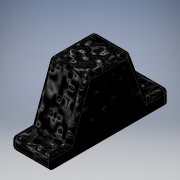
# Autodesk Inventor part: Fuse Block
Saved by Autodesk Inventor 2017 (Build 210142000, 142)
## iProperties
Created: 2017-02-10
Part Number: Fuse Block
Material: Generic
Document SubType Name: Modeling
Designer: michael
Density: 1 g/cm^3
Appearance: Default
Author: michael
Autodesk Inventor part; units mm, degrees
ref_plane "YZ Plane" through (0, 0, 0) normal (1, 0, 0) x (0, 1, 0)
ref_plane "XZ Plane" through (0, 0, 0) normal (0, 1, 0) x (-1, 0, 0)
ref_plane "XY Plane" through (0, 0, 0) normal (0, 0, 1) x (1, 0, 0)
sketch "Sketch1" plane through (0, 0, 0) normal (0, 1, 0) x (-1, 0, 0)
  line L0 (-14.45, 46.075) -> (14.45, 46.075)
  line L1 (14.45, 46.075) -> (14.45, -46.075)
  line L2 (14.45, -46.075) -> (-14.45, -46.075)
  line L3 (-14.45, -46.075) -> (-14.45, 46.075)
  line L4 (-14.45, 46.075) -> (14.45, -46.075) construction
  line L5 (14.45, 46.075) -> (-14.45, -46.075) construction
  point P0 (0, 0)
  dimension "d0" = 28.9
  dimension "d1" = 92.15
  constraints: 12 end point, 2 midpoint, 2 parallel, 1 horizontal, 1 perpendicular
  measures "d0" distance of L1.end L2.end
  measures "d1" distance of L0.end L1.end
extrude "Extrusion1" add sketch "Sketch1" against normal blind 10
sketch "Sketch2" plane through (0, 0, 0) normal (0, 1, 0) x (1, 0, 0)
  point P0 (0, 0)
sketch "Sketch3" plane through (0, 0, 0) normal (0, 1, 0) x (1, 0, 0)
  line L0 (-14.45, -30.5) -> (14.45, -30.5)
  line L1 (14.45, -30.5) -> (14.45, 30.5)
  line L2 (14.45, 30.5) -> (-14.45, 30.5)
  line L3 (-14.45, 30.5) -> (-14.45, -30.5)
  line L4 (-14.45, -30.5) -> (14.45, 30.5) construction
  line L5 (14.45, -30.5) -> (-14.45, 30.5) construction
  point P0 (0, 0)
  dimension "d4" = 28.9
  dimension "d5" = 61
  constraints: 12 end point, 2 midpoint, 2 parallel, 1 horizontal, 1 perpendicular
  measures "d4" distance of L2.end L1.end
  measures "d5" distance of L1.end L0.end
extrude "Extrusion2" add sketch "Sketch3" along normal blind 38
sketch "Sketch4" plane through (0, -10, 0) normal (0, -1, 0) x (1, 0, 0)
  circle A0 centre (0, 39.725) radius 2.7
  circle A1 centre (0, -39.725) radius 2.7
  line L0 (-14.45, -46.075) -> (14.45, -46.075) projected
  line L1 (14.45, -46.075) -> (14.45, 46.075) projected
  point P0 (0, 0)
  dimension "d8" = 5.4
  dimension "d9" = 5.4
  dimension "d10" = 79.45
  dimension "d11" = 6.35
  dimension "d12" = 14.45
  dimension "d13" = 14.45
  constraints: 2 centre point
  measures "d8" diameter of A0
  measures "d9" diameter of A1
  measures "d10" distance of A1.centre A0.centre
  measures "d11" distance from line of L0 A1.centre
  measures "d12" distance from line of L1 A1.centre
  measures "d13" distance from line of L1 A0.centre
hole "Hole1" at (0, -10, -39.725) at (0, -10, 39.725) direction (0, 1, 0) diameter 6.35 end through all
draft "FaceDraft1" angle 20 pull direction (0, 1, 0) faces at (4.8167, 12.6667, -30.5) fixed edges at (0, 0, -30.5)
draft "FaceDraft2" angle 20 pull direction (0, 1, 0) faces at (-4.8167, 12.6667, 30.5) fixed edges at (0, 0, 30.5)
fillet "Fillet1" radius 3.175 19 edges at (14.45, 19, 23.5846) (0, 38, 16.6691) (-14.45, 19, 23.5846) (-14.45, 38, 0) (-14.45, 19, -23.5846) (14.45, 19, -23.5846) (0, 38, -16.6691) (14.45, 38, 0) (14.45, 0, 38.2875) (0, 0, 46.075) (-14.45, 0, 38.2875) (0, -10, 46.075) (-14.45, -5, 46.075) (14.45, -5, -46.075) (14.45, 0, -38.2875) (0, 0, -46.075) (-14.45, 0, -38.2875) (-14.45, -5, -46.075) (-14.45, -10, 0)
equation "\"d13\" = d12"
body "Solid1"
